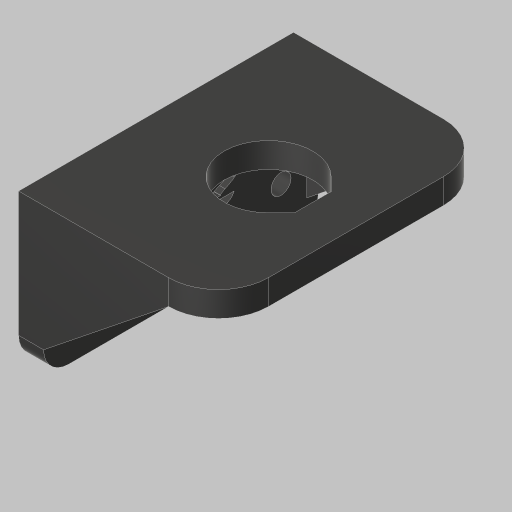
# Autodesk Inventor part: rsl mount
Saved by Autodesk Inventor 2023.5 (Build 275446000, 446)
## iProperties
Created: 2025-02-28
Part Number: rsl mount
Material: ABS Plastic
Document SubType Name: Modeling
Designer: brand
Density: 1.06 g/cm^3
Appearance: Smooth - Black
Author: brand
Autodesk Inventor part; units mm, degrees
ref_plane "YZ Plane" through (0, 0, 0) normal (1, 0, 0) x (0, 1, 0)
ref_plane "XZ Plane" through (0, 0, 0) normal (0, 1, 0) x (-1, 0, 0)
ref_plane "XY Plane" through (0, 0, 0) normal (0, 0, 1) x (1, 0, 0)
sketch "Sketch1" plane through (0, 0, 0) normal (0, 0, 1) x (1, 0, 0)
  line L0 (0, 0) -> (50.8, 0)
  line L1 (50.8, 0) -> (50.8, -6.35)
  line L2 (50.8, -6.35) -> (6.35, -6.35)
  line L3 (6.35, -6.35) -> (6.35, -38.1)
  line L4 (6.35, -38.1) -> (0, -38.1)
  line L5 (0, -38.1) -> (0, 0)
  dimension "d0" = 50.8
  dimension "d1" = 38.1
  dimension "d2" = 6.35
  dimension "d3" = 6.35
  constraints: 12 end point, 5 perpendicular, 1 horizontal
  measures "d0" distance of L0.start L0.end
  measures "d1" distance of L4.end L0.start
  measures "d2" distance of L0.end L1.end
  measures "d3" distance of L3.end L4.end
extrude "Extrusion1" add sketch "Sketch1" along normal mid plane 69.85
sketch "Sketch2" plane through (0, 0, 34.925) normal (0, 1, 0) x (1, 0, 0)
  line L0 (0, 69.85) -> (0, 0) construction
  line L1 (50.8, 0) -> (0, 0) construction
  line L2 (50.8, 69.85) -> (50.8, 0) construction
  line L3 (0, 69.85) -> (50.8, 69.85) construction
  circle A0 centre (28.575, 34.925) radius 11.2522
  line L4 (0, 0) -> (0, 69.85) construction
  line L5 (6.35, 69.85) -> (6.35, 0) construction
  line L6 (6.35, 69.85) -> (6.35, 0) construction
  line L7 (6.35, 69.85) -> (6.35, 0) construction
  line L8 (6.35, 69.85) -> (50.8, 69.85) construction
  line L9 (41.525, 36.525) -> (41.525, 33.325) construction
  line L10 (41.525, 36.525) -> (39.7129, 36.525) construction
  line L11 (41.525, 33.325) -> (39.7129, 33.325) construction
  line L12 (36.5315, 26.9685) -> (44.488, 34.925)
  line L13 (44.488, 34.925) -> (36.5315, 42.8815)
  line L14 (36.5315, 42.8815) -> (39.8272, 42.8815)
  line L15 (39.8272, 42.8815) -> (39.8272, 26.9685)
  line L16 (39.8272, 26.9685) -> (36.5315, 26.9685)
  line L17 (36.5315, 26.9685) -> (36.5315, 42.8815) construction
  point P0 (0, 34.925)
  point P1 (0, 34.925)
  point P2 (28.575, 69.85)
  point P3 (41.525, 34.925)
  point P4 (39.8272, 34.925)
  point P5 (39.8272, 39.5858)
  point P6 (39.8272, 30.2642)
  dimension "d6" = 22.5044
  dimension "d16" = 3.2
  dimension "d17" = 12.95
  constraints: 20 end point, 4 point on circle, 3 horizontal, 3 horizontal alignment, 3 midpoint, 3 perpendicular, 3 tangent, 2 parallel, 1 centre point, 1 vertical, 1 vertical alignment
  measures "d6" diameter of A0
  measures "d16" distance of L9.start L9.end
  measures "d17" distance from line of L9 A0.centre
sketch "Sketch3" plane through (0, -38.1, 34.925) normal (-1, 0, 0) x (0, 0, 1)
  line L0 (0, 0) -> (-69.85, 0) construction
  line L1 (0, 38.1) -> (0, 0) construction
  line L2 (-69.85, 38.1) -> (0, 38.1) construction
  line L3 (-69.85, 0) -> (-69.85, 38.1) construction
  line L4 (-9.525, 25.4) -> (-60.325, 25.4) construction
  line L5 (-60.325, 25.4) -> (-60.325, 12.7) construction
  line L6 (-60.325, 12.7) -> (-9.525, 12.7) construction
  line L7 (-9.525, 12.7) -> (-9.525, 25.4) construction
  line L8 (-9.525, 25.4) -> (-60.325, 12.7) construction
  line L9 (-60.325, 25.4) -> (-9.525, 12.7) construction
  point P0 (-34.925, 38.1)
  point P1 (-34.925, 19.05)
  point P2 (-34.925, 38.1)
  point P3 (0, 19.05)
  dimension "d7" = 50.8
  dimension "d8" = 12.7
  constraints: 12 end point, 4 coincident, 4 midpoint, 2 parallel, 1 horizontal, 1 horizontal alignment, 1 perpendicular, 1 vertical alignment
  measures "d7" distance of L5.end L6.end
  measures "d8" distance of L4.end L5.end
hole "Hole1" at (0, -12.7, -25.4) at (0, -25.4, -25.4) at (0, -25.4, 25.4) at (0, -12.7, 25.4) direction (1, 0, 0) diameter 5.1054 end through all clearance for "Flat Head Machine Screw (82)" size "#10" standard "Ansi Unified Screw Threads"
extrude "Extrusion2" cut sketch "Sketch2" against normal through all contours A0 | L15 L12 A0 | A0 L13 L15
fillet "Fillet1" [suppressed]
fillet "Fillet2" radius 12.7 2 edges at (50.8, -3.175, -34.925) (50.8, -3.175, 34.925)
fillet "Fillet3" radius 6.35 2 edges at (3.175, -38.1, -34.925) (3.175, -38.1, 34.925)
sketch "Sketch5" plane through (0, 0, -34.925) normal (0, 0, -1) x (-1, 0, 0)
  line L0 (0, -31.75) -> (-6.35, -31.75) construction
  line L1 (0, -31.75) -> (0, 0) construction
  line L2 (0, 0) -> (-38.1, 0) construction
  line L3 (-38.1, -6.35) -> (-38.1, 0) construction
  line L4 (-38.1, -6.35) -> (-6.35, -6.35) construction
  line L5 (-6.35, -6.35) -> (-6.35, -31.75) construction
  line L6 (-38.1, -6.35) -> (-6.35, -31.75)
  line L7 (-6.35, -6.35) -> (-6.35, -31.75)
  line L8 (-6.35, -27.9527) -> (-6.35, -22.8473) construction
  line L9 (-6.35, -6.35) -> (-38.1, -6.35)
  line L10 (-17.3228, -6.35) -> (-17.3228, -6.35) construction
  point P0 (-36.5315, -6.35)
  constraints: 6 end point, 2 collinear
extrude "Extrusion3" add sketch "Sketch5" against normal blind 3
mirror "Mirror1" about plane through (0, 0, 0) normal (0, 0, 1) of "Extrusion3"
fillet "Fillet4" radius 6.35 2 edges at (22.225, -6.35, 31.925) (22.225, -6.35, -31.925)
sketch "Sketch6" plane through (6.35, -38.1, 28.575) normal (1, 0, 0) x (0, 0, -1)
  line L0 (43.4887, 15.24) -> (13.6613, 15.24) construction
  line L1 (13.6613, 15.24) -> (13.6613, 22.86) construction
  line L2 (13.6613, 22.86) -> (43.4887, 22.86) construction
  line L3 (43.4887, 22.86) -> (43.4887, 15.24) construction
  line L4 (50.8, 38.1) -> (6.35, 38.1) construction
  circle A0 centre (3.175, 25.4) radius 2.5527 construction
  circle A1 centre (3.175, 12.7) radius 2.5527 construction
  line L5 (3.175, 25.4) -> (3.175, 12.7) construction
  line L6 (43.6281, 22.8842) -> (37.2569, 22.8721)
  line L7 (37.2569, 22.8721) -> (36.7234, 20.9929)
  line L8 (36.7234, 20.9929) -> (39.9303, 20.9929)
  spline S0 degree 2 poles (39.9303, 20.9929) (39.4695, 20.6049) (37.269, 19.7502) (36.8144, 19.4107) knots 0 0 0 1 2 2 2
  spline S1 degree 2 poles (36.8144, 19.4107) (36.0263, 18.7924) (35.8202, 17.8164) knots 0 0 0 1 1 1
  line L9 (35.8202, 17.8164) -> (38.6148, 17.8164)
  spline S2 degree 2 poles (38.6148, 17.8164) (38.6027, 17.8406) (38.6027, 17.8709) knots 0 0 0 1 1 1
  spline S3 degree 2 poles (38.6027, 17.8709) (38.6027, 18.1801) (39.7545, 18.7257) knots 0 0 0 1 1 1
  spline S4 degree 2 poles (39.7545, 18.7257) (41.4579, 19.5198) (42.155, 20.1078) knots 0 0 0 1 1 1
  spline S5 degree 2 poles (42.155, 20.1078) (43.519, 21.2354) (43.6281, 22.8842) knots 0 0 0 1 1 1
  spline S6 degree 2 poles (35.7293, 17.0768) (35.7293, 16.3918) (35.9475, 16.0038) knots 0 0 0 1 1 1
  spline S7 degree 2 poles (35.9475, 16.0038) (36.3718, 15.24) (37.0023, 15.24) knots 0 0 0 1 1 1
  line L10 (37.0023, 15.24) -> (39.712, 15.24)
  spline S8 degree 2 poles (39.712, 15.24) (40.4395, 15.24) (41.8034, 16.3554) (42.0459, 17.0768) knots 0 0 0 1 2 2 2
  line L11 (42.0459, 17.0768) -> (35.7293, 17.0768)
  line L12 (36.3355, 22.8842) -> (29.9642, 22.8721)
  line L13 (29.9642, 22.8721) -> (29.4308, 20.9929)
  line L14 (29.4308, 20.9929) -> (32.6376, 20.9929)
  spline S9 degree 2 poles (32.6376, 20.9929) (32.1769, 20.6049) (29.9764, 19.7502) (29.5217, 19.4107) knots 0 0 0 1 2 2 2
  spline S10 degree 2 poles (29.5217, 19.4107) (28.7337, 18.7924) (28.5275, 17.8164) knots 0 0 0 1 1 1
  line L15 (28.5275, 17.8164) -> (31.3221, 17.8164)
  spline S11 degree 2 poles (31.3221, 17.8164) (31.31, 17.8406) (31.31, 17.8709) knots 0 0 0 1 1 1
  spline S12 degree 2 poles (31.31, 17.8709) (31.31, 18.1801) (32.4618, 18.7257) knots 0 0 0 1 1 1
  spline S13 degree 2 poles (32.4618, 18.7257) (34.1653, 19.5198) (34.8624, 20.1078) knots 0 0 0 1 1 1
  spline S14 degree 2 poles (34.8624, 20.1078) (36.2263, 21.2354) (36.3355, 22.8842) knots 0 0 0 1 1 1
  spline S15 degree 2 poles (28.4366, 17.0768) (28.4366, 16.3918) (28.6548, 16.0038) knots 0 0 0 1 1 1
  spline S16 degree 2 poles (28.6548, 16.0038) (29.0792, 15.24) (29.7096, 15.24) knots 0 0 0 1 1 1
  line L16 (29.7096, 15.24) -> (32.4194, 15.24)
  spline S17 degree 2 poles (32.4194, 15.24) (33.1468, 15.24) (34.5108, 16.3554) (34.7533, 17.0768) knots 0 0 0 1 2 2 2
  line L17 (34.7533, 17.0768) -> (28.4366, 17.0768)
  spline S18 degree 2 poles (25.1874, 19.7865) (24.7266, 19.7865) (24.5387, 19.829) knots 0 0 0 1 1 1
  spline S19 degree 2 poles (24.5387, 19.829) (24.1386, 19.932) (24.1386, 20.2533) knots 0 0 0 1 1 1
  spline S20 degree 2 poles (24.1386, 20.2533) (24.1386, 20.5625) (24.5933, 21.0474) (24.9146, 21.0717) knots 0 0 0 1 2 2 2
  spline S21 degree 2 poles (24.9146, 21.0717) (25.1449, 21.0899) (25.2783, 21.0899) knots 0 0 0 1 1 1
  spline S22 degree 2 poles (25.2783, 21.0899) (25.9209, 21.0899) (25.9209, 20.6837) knots 0 0 0 1 1 1
  spline S23 degree 2 poles (25.9209, 20.6837) (25.9209, 20.6049) (25.9087, 20.5261) knots 0 0 0 1 1 1
  line L18 (25.9087, 20.5261) -> (28.3881, 20.5261)
  spline S24 degree 2 poles (28.3881, 20.5261) (28.4972, 21.2232) (28.4427, 21.4718) knots 0 0 0 1 1 1
  spline S25 degree 2 poles (28.4427, 21.4718) (28.1578, 22.8842) (26.5816, 22.8842) knots 0 0 0 1 1 1
  line L19 (26.5816, 22.8842) -> (24.4053, 22.8842)
  spline S26 degree 2 poles (24.4053, 22.8842) (23.9083, 22.8054) (23.3324, 22.4417) knots 0 0 0 1 1 1
  spline S27 degree 2 poles (23.3324, 22.4417) (22.8231, 22.1204) (22.5928, 21.8234) knots 0 0 0 1 1 1
  spline S28 degree 2 poles (22.5928, 21.8234) (22.0169, 21.0778) (21.8957, 20.126) knots 0 0 0 1 1 1
  spline S29 degree 2 poles (21.8957, 20.126) (21.8835, 19.9987) (21.8835, 19.8775) knots 0 0 0 1 1 1
  spline S30 degree 2 poles (21.8835, 19.8775) (21.8835, 19.2106) (22.2351, 18.7802) knots 0 0 0 1 1 1
  spline S31 degree 2 poles (22.2351, 18.7802) (22.6595, 18.2286) (23.7749, 17.8164) (24.5811, 17.8164) knots 0 0 0 1 2 2 2
  line L20 (24.5811, 17.8164) -> (27.5879, 17.8164)
  line L21 (27.5879, 17.8164) -> (28.1578, 19.7865)
  line L22 (28.1578, 19.7865) -> (25.1874, 19.7865)
  line L23 (21.4956, 17.0768) -> (28.0971, 17.0768)
  line L24 (28.0971, 17.0768) -> (26.9272, 15.24)
  line L25 (26.9272, 15.24) -> (20.9439, 15.24)
  line L26 (20.9439, 15.24) -> (21.4956, 17.0768)
  line L27 (21.6047, 22.8842) -> (15.2335, 22.8721)
  line L28 (15.2335, 22.8721) -> (14.7, 20.9929)
  line L29 (14.7, 20.9929) -> (17.9068, 20.9929)
  spline S32 degree 2 poles (17.9068, 20.9929) (17.4461, 20.6049) (15.2456, 19.7502) (14.7909, 19.4107) knots 0 0 0 1 2 2 2
  spline S33 degree 2 poles (14.7909, 19.4107) (14.0029, 18.7924) (13.7968, 17.8164) knots 0 0 0 1 1 1
  line L30 (13.7968, 17.8164) -> (16.5914, 17.8164)
  spline S34 degree 2 poles (16.5914, 17.8164) (16.5792, 17.8406) (16.5792, 17.8709) knots 0 0 0 1 1 1
  spline S35 degree 2 poles (16.5792, 17.8709) (16.5792, 18.1801) (17.731, 18.7257) knots 0 0 0 1 1 1
  spline S36 degree 2 poles (17.731, 18.7257) (19.4345, 19.5198) (20.1316, 20.1078) knots 0 0 0 1 1 1
  spline S37 degree 2 poles (20.1316, 20.1078) (21.4956, 21.2354) (21.6047, 22.8842) knots 0 0 0 1 1 1
  spline S38 degree 2 poles (13.7058, 17.0768) (13.7058, 16.3918) (13.9241, 16.0038) knots 0 0 0 1 1 1
  spline S39 degree 2 poles (13.9241, 16.0038) (14.3484, 15.24) (14.9789, 15.24) knots 0 0 0 1 1 1
  line L31 (14.9789, 15.24) -> (17.6886, 15.24)
  spline S40 degree 2 poles (17.6886, 15.24) (18.416, 15.24) (19.78, 16.3554) (20.0225, 17.0768) knots 0 0 0 1 2 2 2
  line L32 (20.0225, 17.0768) -> (13.7058, 17.0768)
  point P0 (28.575, 38.1)
  point P1 (28.575, 15.24)
  point P2 (28.575, 38.1)
  point P3 (43.4887, 19.05)
  point P4 (3.175, 19.05)
  point P5 (13.6613, 19.05)
  point P6 (28.575, 22.86)
  point P7 (28.575, 38.1)
  dimension "d0" = 50.8
  dimension "d1" = 38.1
  dimension "d2" = 6.35
  dimension "d3" = 6.35
  dimension "d29" = 7.62
  dimension "d30" = 29.8274
  constraints: 7 midpoint, 2 end point, 1 horizontal, 1 horizontal alignment, 1 vertical, 1 vertical alignment, 2 other
  measures "d29" distance of L2.end L0.start
  measures "d30" distance of L0.start L0.end
extrude "Extrusion4" cut sketch "Sketch6" against normal through all
body "Solid1"
